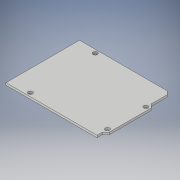
# Autodesk Inventor part: Arduino-Uno-r3
Saved by Autodesk Inventor 2017 (Build 210142000, 142)
## iProperties
Created: 2018-04-18
Part Number: Arduino-Uno-r3
Material: Generic
Document SubType Name: Modeling
Designer: MtgSaber
Density: 1 g/cm^3
Appearance: Default
Author: MtgSaber
Autodesk Inventor part; units mm, degrees
ref_plane "YZ Plane" through (0, 0, 0) normal (1, 0, 0) x (0, 1, 0)
ref_plane "XZ Plane" through (0, 0, 0) normal (0, 1, 0) x (-1, 0, 0)
ref_plane "XY Plane" through (0, 0, 0) normal (0, 0, 1) x (1, 0, 0)
sketch "Sketch1" plane through (0, 0, 0) normal (0, 1, 0) x (-1, 0, 0)
  line L0 (34.29, 26.67) -> (-34.29, 26.67) construction
  line L1 (-34.29, 26.67) -> (-34.29, -26.67) construction
  line L2 (-34.29, -26.67) -> (34.29, -26.67) construction
  line L3 (34.29, -26.67) -> (34.29, 26.67) construction
  line L4 (48.006, 0) -> (-48.006, 0) construction
  line L5 (0, -37.338) -> (0, 37.338) construction
  line L6 (-31.75, -24.13) -> (-31.75, -12.7)
  line L7 (-31.75, 26.67) -> (-31.75, 22.86)
  line L8 (-34.29, -10.16) -> (-34.29, 20.32)
  line L9 (-31.75, -12.7) -> (-31.75, -12.7)
  line L10 (-31.75, 22.86) -> (-31.75, 22.86)
  line L11 (-29.21, -26.67) -> (34.29, -26.67)
  line L12 (34.29, -26.67) -> (34.29, 26.67)
  line L13 (34.29, 26.67) -> (-31.75, 26.67)
  line L14 (-31.75, -24.13) -> (-29.21, -26.67)
  line L15 (-34.29, -10.16) -> (-31.75, -12.7)
  line L16 (-34.29, 20.32) -> (-31.75, 22.86)
  circle A0 centre (20.32, -24.13) radius 1.5875
  circle A1 centre (19.05, 24.13) radius 1.5875
  circle A2 centre (-31.75, 19.05) radius 1.5875
  circle A3 centre (-31.75, -8.89) radius 1.5875
  point P0 (0, 0)
  point P1 (0, -26.67)
  point P2 (-34.29, 0)
  point P3 (-31.75, -26.67)
  point P4 (-34.29, -12.7)
  point P5 (-34.29, 22.86)
  dimension "d0" = 68.58
  dimension "d1" = 53.34
  dimension "d2" = 2.54
  dimension "d3" = 3.81
  dimension "d4" = 13.97
  dimension "d5" = 2.54
  dimension "d6" = 2.54
  dimension "d7" = 2.54
  dimension "d8" = 2.54
  dimension "d9" = 2.54
  dimension "d10" = 2.54
  dimension "d11" = 3.175
  dimension "d12" = 13.97
  dimension "d13" = 15.24
  dimension "d14" = 66.04
  dimension "d15" = 66.04
  dimension "d16" = 27.94
  dimension "d17" = 15.24
  dimension "d18" = 7.62
  dimension "d19" = 2.54
  constraints: 30 end point, 12 point on line, 4 centre point, 3 collinear, 3 equal radius, 3 horizontal, 3 perpendicular, 2 midpoint, 2 parallel, 1 vertical
  measures "d0" distance of L1.end L2.end
  measures "d1" distance of L2.end L0.start
  measures "d2" distance between parallel lines of L1 L6
  measures "d3" distance of L0.end point (-34.29, 22.86)
  measures "d4" distance between parallel lines of L9 L2
  measures "d5" distance of L6.start point (-31.75, -26.67)
  measures "d6" distance of L11.start point (-31.75, -26.67)
  measures "d7" distance of L8.start point (-34.29, -12.7)
  measures "d8" distance of L9.end point (-34.29, -12.7)
  measures "d9" distance of L8.end point (-34.29, 22.86)
  measures "d10" distance of L10.end point (-34.29, 22.86)
  measures "d11" diameter of A0
  measures "d12" horizontal distance of L2.end A0.centre
  measures "d13" horizontal distance of L0.start A1.centre
  measures "d14" horizontal distance of L2.end A3.centre
  measures "d15" distance from line of L3 A2.centre
  measures "d16" distance of A2.centre A3.centre
  measures "d17" vertical distance of A3.centre A0.centre
  measures "d18" distance of L7.start A2.centre
  measures "d19" vertical distance of L0.start A1.centre
extrude "Extrusion1" add sketch "Sketch1" along normal blind 1.6002
equation "\"d6\" = d5"
equation "\"d8\" = d7"
equation "\"d10\" = d9"
body "Solid1"
